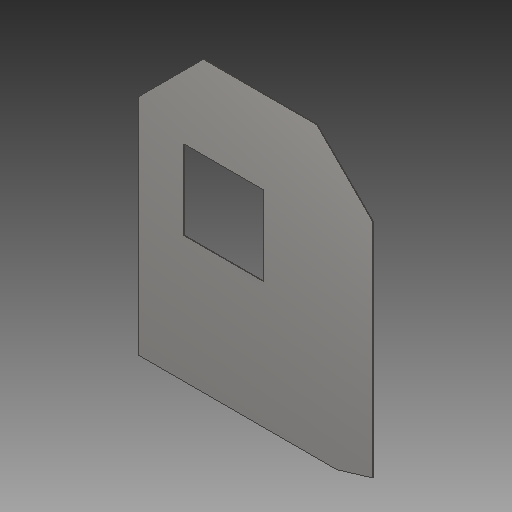
# Autodesk Inventor part: side plate
Saved by Autodesk Inventor 2018 (Build 220112000, 112)
## iProperties
Created: 2018-06-19
Part Number: side plate
Material: Stainless Steel
Document SubType Name: Modeling
Designer: P446509
Density: 8 g/cm^3
Appearance: Stainless - Brushed
Author: P446509
Autodesk Inventor part; units mm, degrees
ref_plane "YZ Plane" through (0, 0, 0) normal (1, 0, 0) x (0, 1, 0)
ref_plane "XZ Plane" through (0, 0, 0) normal (0, 1, 0) x (-1, 0, 0)
ref_plane "XY Plane" through (0, 0, 0) normal (0, 0, 1) x (1, 0, 0)
sketch "Sketch1" plane through (0, 0, 0) normal (0, 0, 1) x (1, 0, 0)
  line L0 (-56, 800) -> (100, 644)
  line L1 (-56, 800) -> (-370, 800)
  line L2 (-314, 350) -> (-204, 350)
  line L3 (-204, 350) -> (-204, 570)
  line L4 (-204, 570) -> (-424, 570)
  line L5 (-424, 570) -> (-424, 350)
  line L6 (-424, 350) -> (-314, 350)
  line L7 (-370, 800) -> (217.6203, 800) construction
  line L8 (0, 0) -> (100, 30)
  line L9 (0, 0) -> (272.914, 0) construction
  line L10 (100, 30) -> (100, 644)
  line L11 (-370, 800) -> (-550, 620)
  line L12 (-370, 800) -> (379.8005, 800) construction
  line L13 (0, 0) -> (-550, 0)
  line L14 (-550, 0) -> (-550, 620)
  dimension "d10" = 110
  dimension "d11" = 220
  dimension "d12" = 220
  dimension "d16" = 800
  dimension "d21" = 100
  dimension "d22" = 135
  dimension "d23" = 135
  dimension "d24" = 550
  dimension "d25" = 126
  dimension "d26" = 230
  dimension "d27" = 314
  dimension "d28" = 180
  dimension "d29" = 30
  constraints: 30 end point, 6 horizontal, 3 perpendicular, 3 vertical
  measures "d10" distance of L2.start L2.end
  measures "d11" distance of L2.end L3.end
  measures "d12" distance of L3.end L4.end
  measures "d16" distance from line of L8.start L1
  measures "d21" distance from line of L8.start L10
  measures "d22" angle of L10 L0
  measures "d23" angle of L11 L12
  measures "d24" distance of L8.start L13.end
  measures "d25" distance between parallel lines of L14 L5
  measures "d26" distance from line of L1.end L4
  measures "d27" distance of L0.start L1.end
  measures "d28" distance from line of L14 L1.end
  measures "d29" distance from line of L13 L8.end
extrude "Extrusion1" add sketch "Sketch1" along normal blind 1.6
body "Solid1"
